Autodesk Inventor part; units mm, degrees
(part 2 of 2)
sketch "Sketch35" plane through (0, 0, 6.35) normal (0, 0, 1) x (1, 0, 0)
  line L0 (289.6654, -107.7256) -> (283.3154, -107.7256)
  line L1 (283.3154, -107.7256) -> (283.3154, -133.1256)
  line L2 (283.3154, -133.1256) -> (289.6654, -133.1256)
  line L3 (289.6654, -133.1256) -> (289.6654, -107.7256)
  point P0 (0, 0)
  dimension "d133" = 6.35
  dimension "d134" = 25.4
  constraints: 8 end point, 2 parallel, 1 horizontal, 1 perpendicular
  measures "d133" distance of L2.end L1.end
  measures "d134" distance of L1.end L0.end
extrude "Extrusion34" cut sketch "Sketch35" against normal blind 25.4
sketch "Sketch36" plane through (0, 0, 6.35) normal (0, 0, 1) x (1, 0, 0)
  line L0 (-24.0246, -568.4816) -> (58.5254, -568.4816)
  line L1 (58.5254, -568.4816) -> (58.5254, -562.1316)
  line L2 (58.5254, -562.1316) -> (-24.0246, -562.1316)
  line L3 (-24.0246, -562.1316) -> (-24.0246, -568.4816)
  point P0 (0, 0)
  constraints: 8 end point, 2 parallel, 1 horizontal, 1 perpendicular
extrude "Extrusion35" add sketch "Sketch36" against normal blind 6.35
sketch "Sketch37" plane through (0, 0, 6.35) normal (0, 0, 1) x (1, 0, 0)
  line L0 (289.6654, -866.9316) -> (164.9006, -866.9316)
  line L1 (164.9006, -866.9316) -> (164.9006, -724.6154)
  line L2 (164.9006, -724.6154) -> (289.6654, -724.6154)
  line L3 (289.6654, -724.6154) -> (289.6654, -866.9316)
  circle A0 centre (164.9006, -724.6154) radius 2.3495
  point P0 (0, 0)
  dimension "d139" = 124.7648
  dimension "d140" = 142.3162
  dimension "d141" = 4.699
  constraints: 8 end point, 2 parallel, 1 centre point, 1 coincident, 1 horizontal, 1 perpendicular
  measures "d139" distance of L1.end L2.end
  measures "d140" distance of L0.end L1.end
  measures "d141" diameter of A0
extrude "Extrusion36" cut sketch "Sketch37" against normal blind 6.35 contours A0 L2 L1 | L1 L2 A0
sketch "Sketch38" plane through (0, 0, 6.35) normal (0, 0, 1) x (1, 0, 0)
  circle A0 centre (164.9006, -724.6154) radius 2.3495 projected
  line L0 (289.6654, -397.0316) -> (289.6654, -133.1256) projected
  line L1 (164.9006, -724.6154) -> (164.9006, -586.9982)
  line L2 (164.9006, -586.9982) -> (164.9006, -368.736)
  circle A1 centre (164.9006, -368.736) radius 2.3495
  circle A2 centre (164.9006, -586.9982) radius 2.3495
  point P0 (0, 0)
  dimension "d144" = 137.6172
  dimension "d145" = 218.2622
  dimension "d146" = 4.699
  dimension "d147" = 4.699
  constraints: 4 end point, 2 centre point, 2 coincident, 1 parallel, 1 point on line
  measures "d144" distance of L1.start L1.end
  measures "d145" distance of L1.end L2.end
  measures "d146" diameter of A1
  measures "d147" diameter of A2
extrude "Extrusion37" cut sketch "Sketch38" against normal blind 6.35 contours A2 L2 L1 | L1 L2 A2 | A1
sketch "Sketch39" plane through (0, 0, 6.35) normal (0, 0, 1) x (1, 0, 0)
  line L0 (289.6654, -133.1256) -> (283.3154, -133.1256) projected
  line L1 (283.3154, -133.1256) -> (283.3154, -107.7256) projected
  line L2 (283.3154, -107.7256) -> (115.9294, -107.7256) projected
  line L3 (115.9294, -107.7256) -> (115.9294, -562.1316) projected
  line L4 (289.6654, -397.0316) -> (289.6654, -133.1256) projected
  line L5 (115.9294, -107.7256) -> (115.9294, -120.4256)
  line L6 (115.9294, -120.4256) -> (283.3154, -120.4256)
  line L7 (283.3154, -133.1256) -> (283.3154, -145.8256)
  line L8 (283.3154, -145.8256) -> (289.6654, -145.8256)
  point P0 (0, 0)
  dimension "d150" = 12.7
  dimension "d151" = 12.7
  constraints: 8 end point, 2 perpendicular, 2 point on line, 1 midpoint
  measures "d150" distance of L2.end L5.end
  measures "d151" distance of L0.end L7.end
extrude "Extrusion38" cut sketch "Sketch39" against normal blind 25.4
sketch "Sketch40" plane through (0, 0, 6.35) normal (0, 0, 1) x (1, 0, 0)
  line L0 (-24.0246, -562.1316) -> (64.8754, -562.1316)
  line L1 (64.8754, -562.1316) -> (64.8754, -568.4816)
  line L2 (64.8754, -568.4816) -> (-24.0246, -568.4816)
  line L3 (-24.0246, -568.4816) -> (-24.0246, -562.1316)
  point P0 (0, 0)
  dimension "d154" = 88.9
  dimension "d155" = 6.35
  constraints: 8 end point, 2 parallel, 1 horizontal, 1 perpendicular
  measures "d154" distance of L1.end L2.end
  measures "d155" distance of L0.end L1.end
extrude "Extrusion39" cut sketch "Sketch40" against normal blind 25.4
sketch "Sketch41" plane through (0, 0, 0) normal (0, 0, -1) x (-1, 0, 0)
  line L0 (24.0246, -568.4816) -> (-64.8754, -568.4816) projected
  line L1 (-64.8754, -568.4816) -> (-39.4754, -568.4816)
  line L2 (-39.4754, -568.4816) -> (-39.4754, -562.1316)
  line L3 (-39.4754, -562.1316) -> (11.3246, -562.1316)
  line L4 (11.3246, -562.1316) -> (11.3246, -568.4816)
  point P0 (0, 0)
  dimension "d158" = 25.4
  dimension "d159" = 50.8
  constraints: 8 end point, 2 perpendicular, 2 point on line, 1 parallel
  measures "d158" distance of L0.end L1.end
  measures "d159" distance of L2.end L3.end
extrude "Extrusion40" add sketch "Sketch41" against normal blind 6.35
body "Solid1"
